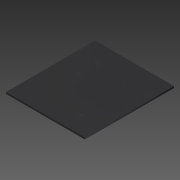
# Autodesk Inventor part: ElectronicsBasePlate
Saved by Autodesk Inventor 2015 (Build 190159000, 159)
## iProperties
Created: 2014-08-22
Part Number: ElectronicsBasePlate
Material: ABS Plastic
Document SubType Name: Modeling
Designer: t_clevj
Density: 1.06 g/cm^3
Appearance: Smooth - Dark Gray
Author: t_clevj
Autodesk Inventor part; units mm, degrees
ref_plane "YZ Plane" through (0, 0, 0) normal (1, 0, 0) x (0, 1, 0)
ref_plane "XZ Plane" through (0, 0, 0) normal (0, 1, 0) x (-1, 0, 0)
ref_plane "XY Plane" through (0, 0, 0) normal (0, 0, 1) x (1, 0, 0)
sketch "Sketch1" plane through (0, 0, 0) normal (0, 0, 1) x (1, 0, 0)
  circle A0 centre (0, 0) radius 1.7295 projected
  line L0 (-10, 9) -> (-10, 3.3) projected
  arc A1 (-10, 3.3) -> (-9.7, 3) centre (-9.7, 3.3) ccw projected
  line L1 (-9.7, 3) -> (-8, 3) projected
  line L2 (-8, 3) -> (-8, 6) projected
  line L3 (-8, 6) -> (-7.0607, 6) projected
  line L4 (-7.0607, 6) -> (-4, 2.9393) projected
  line L5 (-4, 2.9393) -> (-4, 0.5196) projected
  line L6 (-4, 0.5196) -> (-3.7, 0) projected
  line L7 (-3.7, 0) -> (-4, -0.5196) projected
  line L8 (-4, -0.5196) -> (-4, -2.9393) projected
  line L9 (-4, -2.9393) -> (-7.0607, -6) projected
  line L10 (-7.0607, -6) -> (-8, -6) projected
  line L11 (-8, -6) -> (-8, -3) projected
  line L12 (-8, -3) -> (-9.7, -3) projected
  arc A2 (-9.7, -3) -> (-10, -3.3) centre (-9.7, -3.3) ccw projected
  line L13 (-10, -3.3) -> (-10, -9) projected
  arc A3 (-10, -9) -> (-9, -10) centre (-9, -9) ccw projected
  line L14 (-9, -10) -> (-3.3, -10) projected
  arc A4 (-3.3, -10) -> (-3, -9.7) centre (-3.3, -9.7) ccw projected
  line L15 (-3, -9.7) -> (-3, -8) projected
  line L16 (-3, -8) -> (-6, -8) projected
  line L17 (-6, -8) -> (-6, -7.0607) projected
  line L18 (-6, -7.0607) -> (-2.9393, -4) projected
  line L19 (-2.9393, -4) -> (-0.5196, -4) projected
  line L20 (-0.5196, -4) -> (0, -3.7) projected
  line L21 (0, -3.7) -> (0.5196, -4) projected
  line L22 (0.5196, -4) -> (2.9393, -4) projected
  line L23 (2.9393, -4) -> (6, -7.0607) projected
  line L24 (6, -7.0607) -> (6, -8) projected
  line L25 (6, -8) -> (3, -8) projected
  line L26 (3, -8) -> (3, -9.7) projected
  arc A5 (3, -9.7) -> (3.3, -10) centre (3.3, -9.7) ccw projected
  line L27 (3.3, -10) -> (9, -10) projected
  arc A6 (9, -10) -> (10, -9) centre (9, -9) ccw projected
  line L28 (10, -9) -> (10, -3.3) projected
  arc A7 (10, -3.3) -> (9.7, -3) centre (9.7, -3.3) ccw projected
  line L29 (9.7, -3) -> (8, -3) projected
  line L30 (8, -3) -> (8, -6) projected
  line L31 (8, -6) -> (7.0606, -6) projected
  line L32 (7.0606, -6) -> (4, -2.9393) projected
  line L33 (4, -2.9393) -> (4, -0.5196) projected
  line L34 (4, -0.5196) -> (3.7, 0) projected
  line L35 (3.7, 0) -> (4, 0.5196) projected
  line L36 (4, 0.5196) -> (4, 2.9393) projected
  line L37 (4, 2.9393) -> (7.0607, 6) projected
  line L38 (7.0607, 6) -> (8, 6) projected
  line L39 (8, 6) -> (8, 3) projected
  line L40 (8, 3) -> (9.7, 3) projected
  arc A8 (9.7, 3) -> (10, 3.3) centre (9.7, 3.3) ccw projected
  line L41 (10, 3.3) -> (10, 9) projected
  arc A9 (10, 9) -> (9, 10) centre (9, 9) ccw projected
  line L42 (9, 10) -> (3.3, 10) projected
  arc A10 (3.3, 10) -> (3, 9.7) centre (3.3, 9.7) ccw projected
  line L43 (3, 9.7) -> (3, 8) projected
  line L44 (3, 8) -> (6, 8) projected
  line L45 (6, 8) -> (6, 7.0607) projected
  line L46 (6, 7.0607) -> (2.9393, 4) projected
  line L47 (2.9393, 4) -> (0.5196, 4) projected
  line L48 (0.5196, 4) -> (0, 3.7) projected
  line L49 (0, 3.7) -> (-0.5196, 4) projected
  line L50 (-0.5196, 4) -> (-2.9394, 4) projected
  line L51 (-2.9394, 4) -> (-6, 7.0606) projected
  line L52 (-6, 7.0606) -> (-6, 8) projected
  line L53 (-6, 8) -> (-3, 8) projected
  line L54 (-3, 8) -> (-3, 9.7) projected
  arc A11 (-3, 9.7) -> (-3.3, 10) centre (-3.3, 9.7) ccw projected
  line L55 (-3.3, 10) -> (-9, 10) projected
  arc A12 (-9, 10) -> (-10, 9) centre (-9, 9) ccw projected
  circle A13 centre (0, -420) radius 1.7295 projected
  line L56 (-9, -430) -> (-3.3, -430) projected
  arc A14 (-3.3, -430) -> (-3, -429.7) centre (-3.3, -429.7) ccw projected
  line L57 (-3, -429.7) -> (-3, -428) projected
  line L58 (-3, -428) -> (-6, -428) projected
  line L59 (-6, -428) -> (-6, -427.0607) projected
  line L60 (-6, -427.0607) -> (-2.9393, -424) projected
  line L61 (-2.9393, -424) -> (-0.5196, -424) projected
  line L62 (-0.5196, -424) -> (0, -423.7) projected
  line L63 (0, -423.7) -> (0.5196, -424) projected
  line L64 (0.5196, -424) -> (2.9393, -424) projected
  line L65 (2.9393, -424) -> (6, -427.0607) projected
  line L66 (6, -427.0607) -> (6, -428) projected
  line L67 (6, -428) -> (3, -428) projected
  line L68 (3, -428) -> (3, -429.7) projected
  arc A15 (3, -429.7) -> (3.3, -430) centre (3.3, -429.7) ccw projected
  line L69 (3.3, -430) -> (9, -430) projected
  arc A16 (9, -430) -> (10, -429) centre (9, -429) ccw projected
  line L70 (10, -429) -> (10, -423.3) projected
  arc A17 (10, -423.3) -> (9.7, -423) centre (9.7, -423.3) ccw projected
  line L71 (9.7, -423) -> (8, -423) projected
  line L72 (8, -423) -> (8, -426) projected
  line L73 (8, -426) -> (7.0607, -426) projected
  line L74 (7.0607, -426) -> (4, -422.9393) projected
  line L75 (4, -422.9393) -> (4, -420.5196) projected
  line L76 (4, -420.5196) -> (3.7, -420) projected
  line L77 (3.7, -420) -> (4, -419.4804) projected
  line L78 (4, -419.4804) -> (4, -417.0607) projected
  line L79 (4, -417.0607) -> (7.0607, -414) projected
  line L80 (7.0607, -414) -> (8, -414) projected
  line L81 (8, -414) -> (8, -417) projected
  line L82 (8, -417) -> (9.7, -417) projected
  arc A18 (9.7, -417) -> (10, -416.7) centre (9.7, -416.7) ccw projected
  line L83 (10, -416.7) -> (10, -411) projected
  arc A19 (10, -411) -> (9, -410) centre (9, -411) ccw projected
  line L84 (9, -410) -> (3.3, -410) projected
  arc A20 (3.3, -410) -> (3, -410.3) centre (3.3, -410.3) ccw projected
  line L85 (3, -410.3) -> (3, -412) projected
  line L86 (3, -412) -> (6, -412) projected
  line L87 (6, -412) -> (6, -412.9394) projected
  line L88 (6, -412.9394) -> (2.9393, -416) projected
  line L89 (2.9393, -416) -> (0.5196, -416) projected
  line L90 (0.5196, -416) -> (0, -416.3) projected
  line L91 (0, -416.3) -> (-0.5196, -416) projected
  line L92 (-0.5196, -416) -> (-2.9393, -416) projected
  line L93 (-2.9393, -416) -> (-6, -412.9393) projected
  line L94 (-6, -412.9393) -> (-6, -412) projected
  line L95 (-6, -412) -> (-3, -412) projected
  line L96 (-3, -412) -> (-3, -410.3) projected
  arc A21 (-3, -410.3) -> (-3.3, -410) centre (-3.3, -410.3) ccw projected
  line L97 (-3.3, -410) -> (-9, -410) projected
  arc A22 (-9, -410) -> (-10, -411) centre (-9, -411) ccw projected
  line L98 (-10, -411) -> (-10, -416.7) projected
  arc A23 (-10, -416.7) -> (-9.7, -417) centre (-9.7, -416.7) ccw projected
  line L99 (-9.7, -417) -> (-8, -417) projected
  line L100 (-8, -417) -> (-8, -414) projected
  line L101 (-8, -414) -> (-7.0607, -414) projected
  line L102 (-7.0607, -414) -> (-4, -417.0607) projected
  line L103 (-4, -417.0607) -> (-4, -419.4804) projected
  line L104 (-4, -419.4804) -> (-3.7, -420) projected
  line L105 (-3.7, -420) -> (-4, -420.5196) projected
  line L106 (-4, -420.5196) -> (-4, -422.9394) projected
  line L107 (-4, -422.9394) -> (-7.0606, -426) projected
  line L108 (-7.0606, -426) -> (-8, -426) projected
  line L109 (-8, -426) -> (-8, -423) projected
  line L110 (-8, -423) -> (-9.7, -423) projected
  arc A24 (-9.7, -423) -> (-10, -423.3) centre (-9.7, -423.3) ccw projected
  line L111 (-10, -423.3) -> (-10, -429) projected
  arc A25 (-10, -429) -> (-9, -430) centre (-9, -429) ccw projected
  circle A26 centre (370, -420) radius 1.7295 projected
  line L112 (380, -429) -> (380, -423.3) projected
  arc A27 (380, -423.3) -> (379.7, -423) centre (379.7, -423.3) ccw projected
  line L113 (379.7, -423) -> (378, -423) projected
  line L114 (378, -423) -> (378, -426) projected
  line L115 (378, -426) -> (377.0607, -426) projected
  line L116 (377.0607, -426) -> (374, -422.9393) projected
  line L117 (374, -422.9393) -> (374, -420.5196) projected
  line L118 (374, -420.5196) -> (373.7, -420) projected
  line L119 (373.7, -420) -> (374, -419.4804) projected
  line L120 (374, -419.4804) -> (374, -417.0607) projected
  line L121 (374, -417.0607) -> (377.0607, -414) projected
  line L122 (377.0607, -414) -> (378, -414) projected
  line L123 (378, -414) -> (378, -417) projected
  line L124 (378, -417) -> (379.7, -417) projected
  arc A28 (379.7, -417) -> (380, -416.7) centre (379.7, -416.7) ccw projected
  line L125 (380, -416.7) -> (380, -411) projected
  arc A29 (380, -411) -> (379, -410) centre (379, -411) ccw projected
  line L126 (379, -410) -> (373.3, -410) projected
  arc A30 (373.3, -410) -> (373, -410.3) centre (373.3, -410.3) ccw projected
  line L127 (373, -410.3) -> (373, -412) projected
  line L128 (373, -412) -> (376, -412) projected
  line L129 (376, -412) -> (376, -412.9393) projected
  line L130 (376, -412.9393) -> (372.9394, -416) projected
  line L131 (372.9394, -416) -> (370.5196, -416) projected
  line L132 (370.5196, -416) -> (370, -416.3) projected
  line L133 (370, -416.3) -> (369.4804, -416) projected
  line L134 (369.4804, -416) -> (367.0607, -416) projected
  line L135 (367.0607, -416) -> (364, -412.9393) projected
  line L136 (364, -412.9393) -> (364, -412) projected
  line L137 (364, -412) -> (367, -412) projected
  line L138 (367, -412) -> (367, -410.3) projected
  arc A31 (367, -410.3) -> (366.7, -410) centre (366.7, -410.3) ccw projected
  line L139 (366.7, -410) -> (361, -410) projected
  arc A32 (361, -410) -> (360, -411) centre (361, -411) ccw projected
  line L140 (360, -411) -> (360, -416.7) projected
  arc A33 (360, -416.7) -> (360.3, -417) centre (360.3, -416.7) ccw projected
  line L141 (360.3, -417) -> (362, -417) projected
  line L142 (362, -417) -> (362, -414) projected
  line L143 (362, -414) -> (362.9394, -414) projected
  line L144 (362.9394, -414) -> (366, -417.0607) projected
  line L145 (366, -417.0607) -> (366, -419.4804) projected
  line L146 (366, -419.4804) -> (366.3, -420) projected
  line L147 (366.3, -420) -> (366, -420.5196) projected
  line L148 (366, -420.5196) -> (366, -422.9393) projected
  line L149 (366, -422.9393) -> (362.9394, -426) projected
  line L150 (362.9394, -426) -> (362, -426) projected
  line L151 (362, -426) -> (362, -423) projected
  line L152 (362, -423) -> (360.3, -423) projected
  arc A34 (360.3, -423) -> (360, -423.3) centre (360.3, -423.3) ccw projected
  line L153 (360, -423.3) -> (360, -429) projected
  arc A35 (360, -429) -> (361, -430) centre (361, -429) ccw projected
  line L154 (361, -430) -> (366.7, -430) projected
  arc A36 (366.7, -430) -> (367, -429.7) centre (366.7, -429.7) ccw projected
  line L155 (367, -429.7) -> (367, -428) projected
  line L156 (367, -428) -> (364, -428) projected
  line L157 (364, -428) -> (364, -427.0607) projected
  line L158 (364, -427.0607) -> (367.0607, -424) projected
  line L159 (367.0607, -424) -> (369.4804, -424) projected
  line L160 (369.4804, -424) -> (370, -423.7) projected
  line L161 (370, -423.7) -> (370.5196, -424) projected
  line L162 (370.5196, -424) -> (372.9394, -424) projected
  line L163 (372.9394, -424) -> (376, -427.0606) projected
  line L164 (376, -427.0606) -> (376, -428) projected
  line L165 (376, -428) -> (373, -428) projected
  line L166 (373, -428) -> (373, -429.7) projected
  arc A37 (373, -429.7) -> (373.3, -430) centre (373.3, -429.7) ccw projected
  line L167 (373.3, -430) -> (379, -430) projected
  arc A38 (379, -430) -> (380, -429) centre (379, -429) ccw projected
  circle A39 centre (370, 0) radius 1.7295 projected
  line L168 (380, -9) -> (380, -3.3) projected
  arc A40 (380, -3.3) -> (379.7, -3) centre (379.7, -3.3) ccw projected
  line L169 (379.7, -3) -> (378, -3) projected
  line L170 (378, -3) -> (378, -6) projected
  line L171 (378, -6) -> (377.0607, -6) projected
  line L172 (377.0607, -6) -> (374, -2.9393) projected
  line L173 (374, -2.9393) -> (374, -0.5196) projected
  line L174 (374, -0.5196) -> (373.7, 0) projected
  line L175 (373.7, 0) -> (374, 0.5196) projected
  line L176 (374, 0.5196) -> (374, 2.9393) projected
  line L177 (374, 2.9393) -> (377.0607, 6) projected
  line L178 (377.0607, 6) -> (378, 6) projected
  line L179 (378, 6) -> (378, 3) projected
  line L180 (378, 3) -> (379.7, 3) projected
  arc A41 (379.7, 3) -> (380, 3.3) centre (379.7, 3.3) ccw projected
  line L181 (380, 3.3) -> (380, 9) projected
  arc A42 (380, 9) -> (379, 10) centre (379, 9) ccw projected
  line L182 (379, 10) -> (373.3, 10) projected
  arc A43 (373.3, 10) -> (373, 9.7) centre (373.3, 9.7) ccw projected
  line L183 (373, 9.7) -> (373, 8) projected
  line L184 (373, 8) -> (376, 8) projected
  line L185 (376, 8) -> (376, 7.0607) projected
  line L186 (376, 7.0607) -> (372.9394, 4) projected
  line L187 (372.9394, 4) -> (370.5196, 4) projected
  line L188 (370.5196, 4) -> (370, 3.7) projected
  line L189 (370, 3.7) -> (369.4804, 4) projected
  line L190 (369.4804, 4) -> (367.0607, 4) projected
  line L191 (367.0607, 4) -> (364, 7.0607) projected
  line L192 (364, 7.0607) -> (364, 8) projected
  line L193 (364, 8) -> (367, 8) projected
  line L194 (367, 8) -> (367, 9.7) projected
  arc A44 (367, 9.7) -> (366.7, 10) centre (366.7, 9.7) ccw projected
  line L195 (366.7, 10) -> (361, 10) projected
  arc A45 (361, 10) -> (360, 9) centre (361, 9) ccw projected
  line L196 (360, 9) -> (360, 3.3) projected
  arc A46 (360, 3.3) -> (360.3, 3) centre (360.3, 3.3) ccw projected
  line L197 (360.3, 3) -> (362, 3) projected
  line L198 (362, 3) -> (362, 6) projected
  line L199 (362, 6) -> (362.9394, 6) projected
  line L200 (362.9394, 6) -> (366, 2.9393) projected
  line L201 (366, 2.9393) -> (366, 0.5196) projected
  line L202 (366, 0.5196) -> (366.3, 0) projected
  line L203 (366.3, 0) -> (366, -0.5196) projected
  line L204 (366, -0.5196) -> (366, -2.9393) projected
  line L205 (366, -2.9393) -> (362.9394, -6) projected
  line L206 (362.9394, -6) -> (362, -6) projected
  line L207 (362, -6) -> (362, -3) projected
  line L208 (362, -3) -> (360.3, -3) projected
  arc A47 (360.3, -3) -> (360, -3.3) centre (360.3, -3.3) ccw projected
  line L209 (360, -3.3) -> (360, -9) projected
  arc A48 (360, -9) -> (361, -10) centre (361, -9) ccw projected
  line L210 (361, -10) -> (366.7, -10) projected
  arc A49 (366.7, -10) -> (367, -9.7) centre (366.7, -9.7) ccw projected
  line L211 (367, -9.7) -> (367, -8) projected
  line L212 (367, -8) -> (364, -8) projected
  line L213 (364, -8) -> (364, -7.0607) projected
  line L214 (364, -7.0607) -> (367.0607, -4) projected
  line L215 (367.0607, -4) -> (369.4804, -4) projected
  line L216 (369.4804, -4) -> (370, -3.7) projected
  line L217 (370, -3.7) -> (370.5196, -4) projected
  line L218 (370.5196, -4) -> (372.9394, -4) projected
  line L219 (372.9394, -4) -> (376, -7.0606) projected
  line L220 (376, -7.0606) -> (376, -8) projected
  line L221 (376, -8) -> (373, -8) projected
  line L222 (373, -8) -> (373, -9.7) projected
  arc A50 (373, -9.7) -> (373.3, -10) centre (373.3, -9.7) ccw projected
  line L223 (373.3, -10) -> (379, -10) projected
  arc A51 (379, -10) -> (380, -9) centre (379, -9) ccw projected
  line L224 (379, 10) -> (-9, 10)
  line L225 (-10, 9) -> (-10, -429)
  line L226 (-9, -430) -> (379, -430)
  line L227 (380, -429) -> (380, 8.9393)
  point P0 (0, 0)
  constraints: 8 end point, 3 collinear, 1 point on line, 1 tangent
extrude "Extrusion1" add sketch "Sketch1" along normal blind 8 contours A0 | A12 L55 A11 L54 L53 L52 L51 L50 L49 L48 L47 L46 L45 L44 L43 A10 L42 A9 L41 A8 L40 L39 L38 L37 L36 L35 L34 L33 L32 L31 L30 L29 A7 L28 A6 L27 A5 L26 L25 L24 L23 L22 L21 L20 L19 L18 L17 L16 L15 A4 L14 A3 L13 A2 L12 L11 L10 L9 L8 L7 L6 L5 L4 L3 L2 L1 A1 L0 | A1 L1 L2 L3 L4 L5 L6 L7 L8 L9 L10 L11 L12 A2 L225 | L224 A10 L43 L44 L45 L46 L47 L48 L49 L50 L51 L52 L53 L54 A11 | A3 L14 A4 L15 L16 L17 L18 L19 L20 L21 L22 L23 L24 L25 L26 A5 L27 A6 L28 A7 L29 L30 L31 L32 L33 L34 L35 L36 L37 L38 L39 L40 A8 L41 A9 L224 A45 L196 A46 L197 L198 L199 L200 L201 L202 L203 L204 L205 L206 L207 L208 A47 L209 A48 L210 A49 L211 L212 L213 L214 L215 L216 L217 L218 L219 L220 L221 L222 A50 L223 A51 L227 A29 L126 A30 L127 L128 L129 L130 L131 L132 L133 L134 L135 L136 L137 L138 A31 L139 A32 L140 A33 L141 L142 L143 L144 L145 L146 L147 L148 L149 L150 L151 L152 A34 L153 A35 L226 A16 L70 A17 L71 L72 L73 L74 L75 L76 L77 L78 L79 L80 L81 L82 A18 L83 A19 L84 A20 L85 L86 L87 L88 L89 L90 L91 L92 L93 L94 L95 L96 A21 L97 A22 L225 | A22 L97 A21 L96 L95 L94 L93 L92 L91 L90 L89 L88 L87 L86 L85 A20 L84 A19 L83 A18 L82 L81 L80 L79 L78 L77 L76 L75 L74 L73 L72 L71 A17 L70 A16 L69 A15 L68 L67 L66 L65 L64 L63 L62 L61 L60 L59 L58 L57 A14 L56 A25 L111 A24 L110 L109 L108 L107 L106 L105 L104 L103 L102 L101 L100 L99 A23 L98 | A23 L99 L100 L101 L102 L103 L104 L105 L106 L107 L108 L109 L110 A24 L225 | L195 A44 L194 L193 L192 L191 L190 L189 L188 L187 L186 L185 L184 L183 A43 L182 A42 L181 A41 L180 L179 L178 L177 L176 L175 L174 L173 L172 L171 L170 L169 A40 L168 A51 L223 A50 L222 L221 L220 L219 L218 L217 L216 L215 L214 L213 L212 L211 A49 L210 A48 L209 A47 L208 L207 L206 L205 L204 L203 L202 L201 L200 L199 L198 L197 A46 L196 A45 | L224 A43 L183 L184 L185 L186 L187 L188 L189 L190 L191 L192 L193 L194 A44 | A14 L57 L58 L59 L60 L61 L62 L63 L64 L65 L66 L67 L68 A15 L226 | L227 A40 L169 L170 L171 L172 L173 L174 L175 L176 L177 L178 L179 L180 A41 | A35 L153 A34 L152 L151 L150 L149 L148 L147 L146 L145 L144 L143 L142 L141 A33 L140 A32 L139 A31 L138 L137 L136 L135 L134 L133 L132 L131 L130 L129 L128 L127 A30 L126 A29 L125 A28 L124 L123 L122 L121 L120 L119 L118 L117 L116 L115 L114 L113 A27 L112 A38 L167 A37 L166 L165 L164 L163 L162 L161 L160 L159 L158 L157 L156 L155 A36 L154 | A36 L155 L156 L157 L158 L159 L160 L161 L162 L163 L164 L165 L166 A37 L226 | L227 A27 L113 L114 L115 L116 L117 L118 L119 L120 L121 L122 L123 L124 A28 | A13 | A26
body "Solid1"
